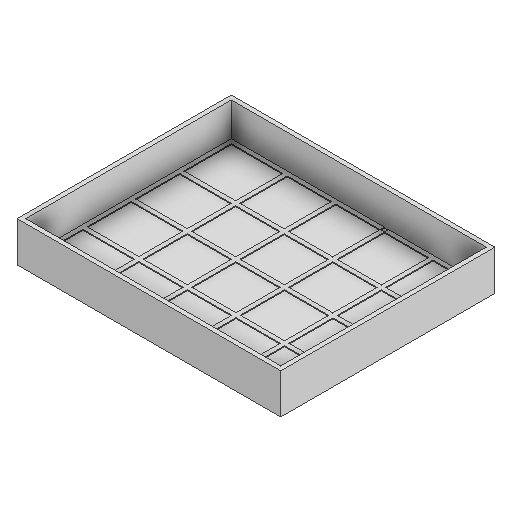
# Autodesk Inventor part: PanHolderLid
Saved by Autodesk Inventor 2025.1 (Build 291241000, 241)
## iProperties
Created: 2025-06-06
Part Number: PanHolderLid
Material: Generic
Document SubType Name: Modeling
Designer: Emlyn
Density: 1 g/cm^3
Appearance: Default
Author: Emlyn
Autodesk Inventor part; units mm, degrees
ref_plane "YZ Plane" through (0, 0, 0) normal (1, 0, 0) x (0, 1, 0)
ref_plane "XZ Plane" through (0, 0, 0) normal (0, 1, 0) x (-1, 0, 0)
ref_plane "XY Plane" through (0, 0, 0) normal (0, 0, 1) x (1, 0, 0)
sketch "Sketch1" plane through (0, 0, 0) normal (0, 1, 0) x (-1, 0, 0)
  line L0 (19.7891, 28.4759) -> (-41.5109, 28.4759)
  line L1 (-41.5109, 28.4759) -> (-41.5109, -21.3241)
  line L2 (-41.5109, -21.3241) -> (19.7891, -21.3241)
  line L3 (19.7891, -21.3241) -> (19.7891, 28.4759)
  point P0 (0, 0)
  dimension "d0" = 49.8
  dimension "d1" = 61.3
  constraints: 8 end point, 2 parallel, 1 horizontal, 1 perpendicular
  measures "d0" distance of L2.end L0.start
  measures "d1" distance of L1.end L2.end
extrude "Extrusion1" add sketch "Sketch1" along normal blind 9.3
sketch "Sketch2" plane through (0, 9.3, 0) normal (0, 1, 0) x (1, 0, 0)
  line L0 (-18.7891, 20.3241) -> (40.5109, 20.3241)
  line L1 (40.5109, 20.3241) -> (40.5109, -27.4759)
  line L2 (40.5109, -27.4759) -> (-18.7891, -27.4759)
  line L3 (-18.7891, -27.4759) -> (-18.7891, 20.3241)
  line L4 (41.5109, 21.3241) -> (-19.7891, 21.3241) projected
  line L5 (-19.7891, 21.3241) -> (-19.7891, -28.4759) projected
  point P0 (0, 0)
  dimension "d4" = 59.3
  dimension "d5" = 47.8
  dimension "d6" = 1
  dimension "d7" = 1
  constraints: 8 end point, 2 parallel, 1 horizontal, 1 perpendicular
  measures "d4" distance of L0.start L0.end
  measures "d5" distance of L2.end L0.start
  measures "d6" distance from line of L4 L0.start
  measures "d7" distance between parallel lines of L5 L3
extrude "Extrusion2" cut sketch "Sketch2" against normal blind 8
sketch "Sketch3" plane through (0, 1.3, 0) normal (0, 1, 0) x (1, 0, 0)
  line L0 (-18.7891, 20.3241) -> (40.5109, 20.3241) projected
  line L1 (40.5109, -27.4759) -> (-18.7891, -27.4759) projected
  line L2 (-18.7891, 20.3241) -> (-17.7891, 20.3241)
  line L3 (-17.7891, 20.3241) -> (-17.7891, -27.4759)
  line L4 (-17.7891, -27.4759) -> (-18.7891, -27.4759)
  line L5 (-18.7891, -27.4759) -> (-18.7891, 20.3241)
  line L6 (-4.7891, 20.3241) -> (-5.7891, 20.3241)
  line L7 (-5.7891, 20.3241) -> (-5.7891, -27.4759)
  line L8 (-5.7891, -27.4759) -> (-4.7891, -27.4759)
  line L9 (-4.7891, -27.4759) -> (-4.7891, 20.3241)
  line L10 (-17.7891, 8.3241) -> (-5.7891, 8.3241)
  line L11 (-5.7891, 8.3241) -> (-5.7891, 7.3241)
  line L12 (-5.7891, 7.3241) -> (-17.7891, 7.3241)
  line L13 (-17.7891, 7.3241) -> (-17.7891, 8.3241)
  line L14 (-17.7891, -2.9259) -> (-5.7891, -2.9259)
  line L15 (-5.7891, -2.9259) -> (-5.7891, -3.9259)
  line L16 (-5.7891, -3.9259) -> (-17.7891, -3.9259)
  line L17 (-17.7891, -3.9259) -> (-17.7891, -2.9259)
  line L18 (-17.7891, -14.1759) -> (-5.7891, -14.1759)
  line L19 (-5.7891, -14.1759) -> (-5.7891, -15.1759)
  line L20 (-5.7891, -15.1759) -> (-17.7891, -15.1759)
  line L21 (-17.7891, -15.1759) -> (-17.7891, -14.1759)
  line L22 (-19.7891, 21.3241) -> (-19.7891, -28.4759) projected
  line L23 (-17.7891, 20.3241) -> (-5.7891, 20.3241)
  line L24 (-5.7891, 20.3241) -> (-5.7891, 19.3241)
  line L25 (-5.7891, 19.3241) -> (-17.7891, 19.3241)
  line L26 (-17.7891, 19.3241) -> (-17.7891, 20.3241)
  line L27 (-17.7891, -26.4759) -> (-5.7891, -26.4759)
  line L28 (-5.7891, -26.4759) -> (-5.7891, -27.4759)
  line L29 (-5.7891, -27.4759) -> (-17.7891, -27.4759)
  line L30 (-17.7891, -27.4759) -> (-17.7891, -26.4759)
  line L31 (5.5109, 19.3241) -> (-6.4891, 19.3241)
  line L32 (6.5109, -27.4759) -> (6.5109, 20.3241)
  line L33 (5.5109, 20.3241) -> (5.5109, -27.4759)
  line L34 (-6.4891, 8.3241) -> (5.5109, 8.3241)
  line L35 (5.5109, 7.3241) -> (-6.4891, 7.3241)
  line L36 (-6.4891, -2.9259) -> (5.5109, -2.9259)
  line L37 (5.5109, -3.9259) -> (-6.4891, -3.9259)
  line L38 (-6.4891, -14.1759) -> (5.5109, -14.1759)
  line L39 (5.5109, -15.1759) -> (-6.4891, -15.1759)
  line L40 (-6.4891, -26.4759) -> (5.5109, -26.4759)
  line L41 (5.5109, -27.4759) -> (-6.4891, -27.4759)
  line L42 (16.8109, 19.3241) -> (4.8109, 19.3241)
  line L43 (17.8109, -27.4759) -> (17.8109, 20.3241)
  line L44 (16.8109, 20.3241) -> (16.8109, -27.4759)
  line L45 (4.8109, 8.3241) -> (16.8109, 8.3241)
  line L46 (16.8109, 7.3241) -> (4.8109, 7.3241)
  line L47 (4.8109, -2.9259) -> (16.8109, -2.9259)
  line L48 (16.8109, -3.9259) -> (4.8109, -3.9259)
  line L49 (4.8109, -14.1759) -> (16.8109, -14.1759)
  line L50 (16.8109, -15.1759) -> (4.8109, -15.1759)
  line L51 (4.8109, -26.4759) -> (16.8109, -26.4759)
  line L52 (16.8109, -27.4759) -> (4.8109, -27.4759)
  line L53 (28.1109, 19.3241) -> (16.1109, 19.3241)
  line L54 (29.1109, -27.4759) -> (29.1109, 20.3241)
  line L55 (28.1109, 20.3241) -> (28.1109, -27.4759)
  line L56 (16.1109, 8.3241) -> (28.1109, 8.3241)
  line L57 (28.1109, 7.3241) -> (16.1109, 7.3241)
  line L58 (16.1109, -2.9259) -> (28.1109, -2.9259)
  line L59 (28.1109, -3.9259) -> (16.1109, -3.9259)
  line L60 (16.1109, -14.1759) -> (28.1109, -14.1759)
  line L61 (28.1109, -15.1759) -> (16.1109, -15.1759)
  line L62 (16.1109, -26.4759) -> (28.1109, -26.4759)
  line L63 (28.1109, -27.4759) -> (16.1109, -27.4759)
  line L64 (39.4109, 19.3241) -> (27.4109, 19.3241)
  line L65 (40.4109, -27.4759) -> (40.4109, 20.3241)
  line L66 (39.4109, 20.3241) -> (39.4109, -27.4759)
  line L67 (27.4109, 8.3241) -> (39.4109, 8.3241)
  line L68 (39.4109, 7.3241) -> (27.4109, 7.3241)
  line L69 (27.4109, -2.9259) -> (39.4109, -2.9259)
  line L70 (39.4109, -3.9259) -> (27.4109, -3.9259)
  line L71 (27.4109, -14.1759) -> (39.4109, -14.1759)
  line L72 (39.4109, -15.1759) -> (27.4109, -15.1759)
  line L73 (27.4109, -26.4759) -> (39.4109, -26.4759)
  line L74 (39.4109, -27.4759) -> (27.4109, -27.4759)
  point P0 (0, 0)
  point P1 (-11.7891, 8.3241)
  point P2 (-0.4891, 8.3241)
  point P3 (10.8109, 8.3241)
  point P4 (22.1109, 8.3241)
  point P5 (33.4109, 8.3241)
  point P6 (-18.7891, -27.4759)
  point P7 (40.4109, 20.3241)
  point P8 (17.8109, 20.3241)
  point P9 (17.8109, 19.3241)
  point P10 (17.8109, 8.3241)
  point P11 (6.5109, 8.3241)
  point P12 (6.5109, 19.3241)
  point P13 (-4.7891, 19.3241)
  point P14 (-4.7891, 8.3241)
  point P15 (-4.7891, 7.3241)
  point P16 (-4.7891, -2.9259)
  point P17 (-4.7891, -3.9259)
  point P18 (-4.7891, -14.1759)
  point P19 (6.5109, -3.9259)
  point P20 (6.5109, -14.1759)
  point P21 (17.8109, 7.3241)
  point P22 (17.8109, -2.9259)
  point P23 (17.8109, -15.1759)
  point P24 (17.8109, -26.4759)
  point P25 (29.1109, -2.9259)
  point P26 (29.1109, 7.3241)
  point P27 (29.1109, -26.4759)
  point P28 (29.1109, -15.1759)
  point P29 (29.1109, -14.1759)
  point P30 (29.1109, -3.9259)
  point P31 (29.1109, 19.3241)
  point P32 (29.1109, 8.3241)
  point P33 (17.8109, -3.9259)
  point P34 (17.8109, -14.1759)
  point P35 (6.5109, -15.1759)
  point P36 (6.5109, -26.4759)
  point P37 (6.5109, 7.3241)
  point P38 (6.5109, -2.9259)
  point P39 (-4.7891, -15.1759)
  point P40 (-4.7891, -26.4759)
  dimension "d10" = 1
  dimension "d12" = 1
  dimension "d13" = 12
  dimension "d14" = 1
  dimension "d15" = 12
  dimension "d16" = 1
  dimension "d17" = 1
  dimension "d18" = 10.25
  dimension "d19" = 10.25
  dimension "d20" = 2
  dimension "d21" = 1
  dimension "d22" = 1
  dimension "d25" = 11.3
  constraints: 144 end point, 28 point on line, 14 parallel, 8 horizontal, 7 perpendicular, 1 midpoint, 132 other
  measures "d10" distance between parallel lines of L3 L5
  measures "d12" distance between parallel lines of L7 L9
  measures "d13" distance between parallel lines of L3 L7
  measures "d14" distance from line of L12 point (-11.789, 8.324)
  measures "d15" distance between parallel lines of L10 L0
  measures "d16" distance between parallel lines of L16 L14
  measures "d17" distance between parallel lines of L20 L18
  measures "d18" distance between parallel lines of L14 L12
  measures "d19" distance between parallel lines of L18 L16
  measures "d20" distance between parallel lines of L22 L3
  measures "d21" distance between parallel lines of L0 L25
  measures "d22" distance between parallel lines of L1 L27
  measures "d25" distance of L24.end L31.start
extrude "Extrusion3" add sketch "Sketch3" along normal blind 0.2 contours L0 L3 L1 L5 | L0 L7 L25 L3 | L0 L9 L31 L7 | L3 L27 L7 L1 | L0 L33 L31 L9 | L31 L9 L34 L7 | L10 L7 L12 L3 | L0 L32 L42 L33 | L34 L9 L35 L7 | L7 L40 L9 L1 | L3 L18 L7 L20 | L0 L44 L42 L32 | L42 L32 L45 L33 | L34 L33 L35 L9 | L35 L9 L36 L7 | L14 L7 L16 L3 | L9 L40 L33 L1 | L7 L39 L9 L40 | L45 L32 L46 L33 | L36 L9 L37 L7 | L7 L38 L9 L39 | L0 L55 L53 L43 | L53 L43 L56 L44 | L45 L44 L46 L32 | L46 L32 L47 L33 | L36 L33 L37 L9 | L37 L9 L38 L7 | L33 L51 L32 L1 | L9 L38 L33 L39 | L0 L54 L64 L55 | L56 L43 L57 L44 | L47 L32 L48 L33 | L32 L51 L44 L1 | L33 L50 L32 L51 | L0 L66 L64 L54 | L64 L54 L67 L55 | L56 L55 L57 L43 | L57 L43 L58 L44 | L47 L44 L48 L32 | L48 L32 L49 L33 | L33 L49 L32 L50 | L0 L65 L1 L66 | L67 L54 L68 L55 | L58 L43 L59 L44 | L44 L62 L43 L1 | L32 L49 L44 L50 | L67 L66 L68 L54 | L68 L54 L69 L55 | L58 L55 L59 L43 | L59 L43 L60 L44 | L43 L62 L55 L1 | L44 L61 L43 L62 | L69 L54 L70 L55 | L60 L43 L61 L44 | L1 L54 L73 L66 | L69 L66 L70 L54 | L70 L54 L71 L55 | L60 L55 L61 L43 | L55 L73 L54 L1 | L71 L54 L72 L55 | L55 L72 L54 L73 | L72 L54 L71 L66
body "Solid1"
